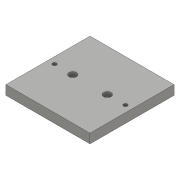
# Autodesk Inventor part: Grundplatte_2016_iLogic
Saved by Autodesk Inventor 2016 (Build 200138000, 138)
## iProperties
Created: 2015-09-07
Part Number: Grundplatte_2016_iLogic
Material: Generisch
Document SubType Name: Modeling
Designer: bauermeisterdi
Density: 1 g/cm^3
Appearance: Vorgabe
Author: bauermeisterdi
Autodesk Inventor part; units mm, degrees
ref_plane "YZ Plane" through (0, 0, 0) normal (1, 0, 0) x (0, 1, 0)
ref_plane "XZ Plane" through (0, 0, 0) normal (0, 1, 0) x (-1, 0, 0)
ref_plane "XY Plane" through (0, 0, 0) normal (0, 0, 1) x (1, 0, 0)
sketch "Skizze_Grundkörper" plane through (0, 0, 0) normal (0, 0, 1) x (1, 0, 0)
  line L0 (-63, 0) -> (63, 0) projected
  line L1 (0, -63) -> (0, 63) projected
  line L2 (45, -45) -> (-45, -45)
  line L3 (-45, -45) -> (-45, 45)
  line L4 (-45, 45) -> (45, 45)
  line L5 (45, 45) -> (45, -45)
  line L6 (45, -45) -> (-45, 45) construction
  line L7 (-45, -45) -> (45, 45) construction
  point P0 (0, 0)
  dimension "Breite" = 90
  dimension "Länge" = 90
  constraints: 12 end point, 2 midpoint, 2 parallel, 1 horizontal, 1 perpendicular
  measures "Breite" distance of L3.end L4.end
  measures "Länge" distance of L2.end L3.end
extrude "Grundkörper" add sketch "Skizze_Grundkörper" along normal mid plane 10
sketch "Skizze_Senkbohrung" plane through (0, 0, 5) normal (0, 0, 1) x (1, 0, 0)
  line L0 (-63, 0) -> (63, 0) projected
  line L1 (0, -63) -> (0, 63) projected
  point P0 (0, 0)
  point P1 (-18.5, 0)
  point P2 (18.5, 0)
  dimension "Senkbohrung_Abstand" = 37
  constraints: 2 point on line, 1 symmetric about line
  measures "Senkbohrung_Abstand" distance of point (18.5, 0) point (-18.5, 0)
hole "Senkbohrung" at (-18.5, 0, 5) at (18.5, 0, 5) direction (0, 0, -1) diameter 4.5 end through all counterbore diameter 8 counterbore depth 4.4
sketch "Skizze_Gewindebohrung_M5" plane through (0, 0, 5) normal (0, 0, 1) x (1, 0, 0)
  line L0 (-63, 0) -> (63, 0) projected
  line L1 (0, -63) -> (0, 63) projected
  point P0 (0, 0)
  point P1 (-38, 0)
  point P2 (38, 0)
  dimension "Gewindeabstand" = 76
  constraints: 2 point on line, 1 symmetric about line
  measures "Gewindeabstand" distance of point (38, 0) point (-38, 0)
hole "Gewindebohrung_M5" at (-38, 0, 5) at (38, 0, 5) direction (0, 0, -1) diameter 4.134 end through all thread size "M5x0.8" class "6H" standard "ISO Metric profile"
